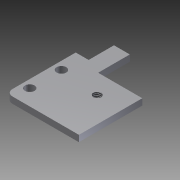
# Autodesk Inventor part: Tope End Stop carroX
Saved by Autodesk Inventor 2015 (Build 190159000, 159)
## iProperties
Created: 2014-06-18
Part Number: Tope End Stop carroX
Document SubType Name: Modeling
Designer: Lorenzo
Density: 1 g/cm^3
Material: Generic
Appearance: Default
Author: Lorenzo
Autodesk Inventor part; units mm, degrees
ref_plane "YZ Plane" through (0, 0, 0) normal (1, 0, 0) x (0, 1, 0)
ref_plane "XZ Plane" through (0, 0, 0) normal (0, 1, 0) x (-1, 0, 0)
ref_plane "XY Plane" through (0, 0, 0) normal (0, 0, 1) x (1, 0, 0)
sketch "Boceto1" plane through (0, 0, 0) normal (0, 0, 1) x (1, 0, 0)
  circle A0 centre (-0.0513, 4.8178) radius 1.2295 projected
  circle A1 centre (-0.0513, -5.1822) radius 1.2295 projected
  line L0 (2.4487, 9.8178) -> (2.4487, -10.1822) projected
  line L1 (-2.5512, 9.8178) -> (2.4487, 9.8178) projected
  line L2 (-2.5512, 9.8178) -> (-2.5512, -8.1822) projected
  arc A2 (-2.5512, -8.1822) -> (-0.5512, -10.1822) centre (-0.5512, -8.1822) ccw projected
  line L3 (-0.5512, -10.1822) -> (2.4487, -10.1822) projected
  line L4 (2.4487, -10.1822) -> (20.4487, -10.1822)
  line L5 (2.4487, 9.8178) -> (20.4487, 9.8178)
  line L6 (20.4487, -10.1822) -> (20.4487, 9.8178)
  line L7 (1.5168, 9.8178) -> (6.5168, 9.8178)
  line L8 (6.5168, 9.8178) -> (6.5168, 19.8178)
  line L9 (6.5168, 19.8178) -> (1.5168, 19.8178)
  line L10 (1.5168, 19.8178) -> (1.5168, 9.8178)
  dimension "d0" = 18
  dimension "d1" = 18
  dimension "d4" = 5
  dimension "d5" = 10
  constraints: 14 end point, 3 parallel, 1 collinear, 1 horizontal, 1 perpendicular, 1 point on line
  measures "d0" distance of L0.start L5.end
  measures "d1" distance of L0.end L4.end
  measures "d4" distance of L8.end L9.end
  measures "d5" distance of L7.end L8.end
extrude "Extrusión1" add sketch "Boceto1" along normal blind 2
sketch "Boceto2" plane through (-2.5512, 9.8178, 0) normal (0, 1, 0) x (1, 0, 0)
  line L0 (4.068, 0) -> (4.068, -2) projected
  line L1 (4.068, 0) -> (0, 0) projected
  line L2 (0, 0) -> (0, -2) projected
  line L3 (0, -2) -> (4.068, -2) projected
extrude "Extrusión2" add sketch "Boceto2" along normal blind 2
sketch "Boceto3" plane through (0, 0, 0) normal (0, 0, -1) x (-1, 0, 0)
  circle A0 centre (-12.4487, 3.608) radius 1.5 projected
hole "Agujero1" at (12.4487, 3.608, 0) direction (0, 0, 1) diameter 2.459 end through all thread size "M3x0.5" class "6H" standard "ISO Metric profile"
sketch "Boceto4" plane through (0, 0, 2) normal (0, 0, 1) x (1, 0, 0)
  circle A0 centre (-0.0513, -5.1822) radius 1.2295 projected
  circle A1 centre (-0.0513, 4.8178) radius 1.2295 projected
  circle A2 centre (-0.0513, 4.8178) radius 1.5
  circle A3 centre (-0.0513, -5.1822) radius 1.5
  dimension "d15" = 3
  dimension "d16" = 3
  constraints: 2 centre point, 2 coincident
  measures "d15" diameter of A2
  measures "d16" diameter of A3
extrude "Extrusión3" cut sketch "Boceto4" against normal up to next
body "Solid1"
